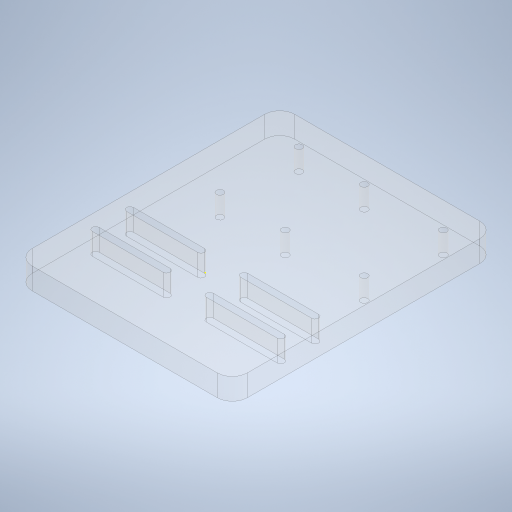
# Autodesk Inventor part: bas
Saved by Autodesk Inventor 2024 (Build 280153000, 153)
## iProperties
Created: 2024-08-11
Part Number: bas
Material: Polycarbonate, Clear
Document SubType Name: Modeling
Designer: drica
Density: 1.2 g/cm^3
Appearance: Polycarbonate - Clear
Author: drica
Autodesk Inventor part; units mm, degrees
ref_plane "YZ Plane" through (0, 0, 0) normal (1, 0, 0) x (0, 1, 0)
ref_plane "XZ Plane" through (0, 0, 0) normal (0, 1, 0) x (-1, 0, 0)
ref_plane "XY Plane" through (0, 0, 0) normal (0, 0, 1) x (1, 0, 0)
sketch "Sketch1" plane through (0, 0, 0) normal (0, 1, 0) x (-1, 0, 0)
  line L0 (50, 37.5) -> (-50, 37.5)
  line L1 (-50, 37.5) -> (-50, -37.5)
  line L2 (-50, -37.5) -> (50, -37.5)
  line L3 (50, -37.5) -> (50, 37.5)
  line L4 (50, 37.5) -> (-50, -37.5) construction
  line L5 (-50, 37.5) -> (50, -37.5) construction
  line L6 (0, 0) -> (-10, 0)
  line L7 (-10, 0) -> (-10, 8)
  line L8 (-10, 0) -> (-2, 0) construction
  line L9 (-10, 0) -> (-10, -8)
  line L10 (-10, 0) -> (-2, 0) construction
  line L11 (-10, 8) -> (-43, 8) construction
  line L12 (-10, 9.6) -> (-43, 9.6)
  line L13 (-43, 6.4) -> (-10, 6.4)
  arc A0 (-10, 6.4) -> (-10, 9.6) centre (-10, 8) ccw
  arc A1 (-43, 9.6) -> (-43, 6.4) centre (-43, 8) ccw
  line L14 (-10, 8) -> (23, 8) construction
  line L15 (0, 0) -> (-50, 0)
  line L16 (-10, -8) -> (-43, -8) construction
  line L17 (-10, -6.4) -> (-43, -6.4)
  line L18 (-43, -9.6) -> (-10, -9.6)
  arc A2 (-10, -9.6) -> (-10, -6.4) centre (-10, -8) ccw
  arc A3 (-43, -6.4) -> (-43, -9.6) centre (-43, -8) ccw
  line L19 (-10, -8) -> (23, -8) construction
  line L20 (0, 37.5) -> (0, -37.5)
  line L21 (10, 0) -> (10, 8)
  line L22 (10, 0) -> (10, -8)
  line L23 (10, 8) -> (43, 8) construction
  line L24 (10, 9.6) -> (43, 9.6)
  line L25 (43, 6.4) -> (10, 6.4)
  arc A4 (10, 9.6) -> (10, 6.4) centre (10, 8) ccw
  arc A5 (43, 6.4) -> (43, 9.6) centre (43, 8) ccw
  line L26 (10, -8) -> (43, -8) construction
  line L27 (10, -6.4) -> (43, -6.4)
  line L28 (43, -9.6) -> (10, -9.6)
  arc A6 (10, -6.4) -> (10, -9.6) centre (10, -8) ccw
  arc A7 (43, -9.6) -> (43, -6.4) centre (43, -8) ccw
  point P0 (-26.5, 8)
  point P1 (-26.5, -8)
  point P2 (26.5, 8)
  point P3 (26.5, -8)
  dimension "d0" = 100
  dimension "d1" = 75
  dimension "d2" = 10
  dimension "d3" = 8
  dimension "d4" = 90
  dimension "d5" = 8
  dimension "d6" = 90
  dimension "d7" = 33
  dimension "d8" = 180
  dimension "d9" = 3.2
  dimension "d10" = 33
  dimension "d11" = 180
  dimension "d12" = 3.2
  constraints: 66 end point, 16 point on circle, 15 symmetric about line, 8 centre point, 8 horizontal, 8 tangent, 7 midpoint, 4 equal length, 4 parallel, 2 vertical, 1 perpendicular, 4 other
  measures "d0" distance of L2.end L1.end
  measures "d1" distance of L1.end L0.end
  measures "d2" distance of L6.start L6.end
  measures "d3" distance of L6.end L7.end
  measures "d4" angle of L8 L7
  measures "d5" distance of L6.end L9.end
  measures "d6" angle of L9 L10
  measures "d7" distance of L7.end L11.end
  measures "d8" angle of L11 L14
  measures "d9" diameter of A1
  measures "d10" distance of L9.end L16.end
  measures "d11" angle of L16 L19
  measures "d12" diameter of A3
extrude "Extrusion1" add sketch "Sketch1" along normal blind 10
sketch "Sketch2" plane through (0, 10, 0) normal (0, 1, 0) x (1, 0, 0)
  line L0 (50, 37.5) -> (-50, 37.5) projected
  line L1 (-50, 37.5) -> (50, 37.5)
  line L2 (50, 37.5) -> (50, 84.5)
  line L3 (50, 84.5) -> (-50, 84.5)
  line L4 (-50, 84.5) -> (-50, 37.5)
  point P0 (0, 0)
  dimension "d15" = 47
  constraints: 8 end point, 2 parallel, 1 horizontal, 1 perpendicular
  measures "d15" distance of L2.end L1.end
extrude "Extrusion2" add sketch "Sketch2" against normal blind 10
sketch "Sketch3" plane through (0, 10, 0) normal (0, 1, 0) x (1, 0, 0)
  line L0 (38.0429, 35.7373) -> (1.3429, 35.7373)
  line L1 (1.3429, 35.7373) -> (1.3429, 72.4373)
  line L2 (1.3429, 72.4373) -> (38.0429, 72.4373)
  line L3 (38.0429, 72.4373) -> (38.0429, 35.7373)
  circle A0 centre (1.3429, 72.4373) radius 1.65
  circle A1 centre (1.3429, 35.7373) radius 1.65
  circle A2 centre (38.0429, 35.7373) radius 1.65
  circle A3 centre (38.0429, 72.4373) radius 1.65
  line L4 (-28.9751, 35.7373) -> (-28.9751, 72.4373)
  circle A4 centre (-28.9751, 72.4373) radius 1.65
  circle A5 centre (-28.9751, 35.7373) radius 1.65
  point P0 (0, 0)
  dimension "d18" = 36.7
  dimension "d19" = 36.7
  dimension "d20" = 3.3
  dimension "d21" = 3.3
  dimension "d22" = 3.3
  dimension "d23" = 3.3
  dimension "d24" = 36.7
  dimension "d25" = 3.3
  dimension "d26" = 3.3
  constraints: 10 end point, 6 centre point, 6 coincident, 2 parallel, 1 horizontal, 1 perpendicular
  measures "d18" distance of L1.end L2.end
  measures "d19" distance of L0.end L1.end
  measures "d20" diameter of A0
  measures "d21" diameter of A1
  measures "d22" diameter of A2
  measures "d23" diameter of A3
  measures "d24" distance of L4.start L4.end
  measures "d25" diameter of A4
  measures "d26" diameter of A5
extrude "Extrusion3" cut sketch "Sketch3" against normal blind 10 contours A1 L1 L0 | L0 L1 A1 | A2 L3 L0 | L0 L3 A2 | A0 L2 L1 | L1 L2 A0 | A3 L2 L3 | L3 L2 A3 | A4 | A5
sketch "Sketch4" plane through (0, 10, 0) normal (0, 1, 0) x (1, 0, 0)
  point P0 (0, 0)
fillet "Fillet1" radius 7 4 edges at (-50, 5, 37.5) (50, 5, 37.5) (50, 5, -84.5) (-50, 5, -84.5)
body "Solid1"
